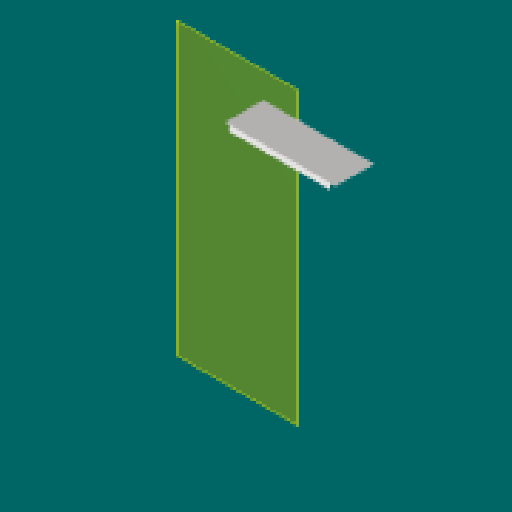
# Autodesk Inventor part: G_S
Saved by Autodesk Inventor 2023 (Build 270158000, 158)
## iProperties
Created: 2023-01-28
Part Number: G_S
Material: Generic
Document SubType Name: Sheet Metal
Designer: HeavyDrewno
Density: 1 g/cm^3
Sheet Metal Rule: Default
Appearance: Default
Author: HeavyDrewno
Autodesk Inventor part; units mm, degrees
ref_plane "YZ Plane" through (0, 0, 0) normal (1, 0, 0) x (0, 1, 0)
ref_plane "XZ Plane" through (0, 0, 0) normal (0, 1, 0) x (-1, 0, 0)
ref_plane "XY Plane" through (0, 0, 0) normal (0, 0, 1) x (1, 0, 0)
ref_plane "Work Plane1" through (0, 0, 0) normal (0, 0, 1) x (1, 0, 0)
sketch "Sketch1" plane through (0, 0, 0) normal (0, 0, 1) x (1, 0, 0)
  line L0 (-196, 470) -> (196, 470) construction
  line L1 (-196, 470) -> (-196, 330) construction
  line L2 (-196, 330) -> (196, 330)
  point P0 (0, 0)
  dimension "d0" = 140
  measures "d0" distance of L0.start L1.end
sketch "Sketch2" plane through (-196, 330, 136) normal (0, 0, 1) x (1, 0, 0)
  line L0 (16, 140) -> (16, -860) construction
  line L1 (376, 140) -> (376, -860) construction
  line L2 (0, 0) -> (392, 0)
  line L3 (16, 0) -> (16, -20)
  line L4 (16, -20) -> (376, -20)
  line L5 (376, -20) -> (376, 0)
  line L6 (16, 0) -> (376, 0)
  point P0 (196, -330)
  dimension "d12" = 20
  measures "d12" distance of L3.start L3.end
contour flange "Contour Flange1" sketch "Sketch1" thickness 2 bend radius 2 width 136 along (0, 0, 1) mid plane no both sides no wall seen from (0, 330, 0) lies toward (0, -1, 0) curves L2
bend "Bend1"
corner "Corner1"
sheet face with bend "Face1" sketch "Sketch2" thickness 2 toward (0, 0, 1) bend radius 2 relief straight relief width 2 relief depth 1
bend "Bend2"
equation "\"d1\" = Thickness"
equation "\"d2\" = BendReliefWidth"
equation "\"d3\" = BendReliefDepth"
equation "\"d4\" = MinimumRemnant"
equation "\"d5\" = TransitionRadius"
equation "\"d7\" = BendRadius"
equation "\"d9\" = CornerReliefSize"
equation "\"d10\" = GapSize"
equation "\"d11\" = JacobiRadiusSize"
equation "\"d13\" = BendRadius"
equation "\"d14\" = BendReliefWidth"
equation "\"d16\" = MinimumRemnant"
equation "\"d15\" = BendReliefDepth"
equation "\"d17\" = TransitionRadius"
equation "\"BendRadius\" = Thickness"
equation "\"BendReliefWidth\" = Thickness"
equation "\"BendReliefDepth\" = 0.5 * Thickness"
equation "\"CornerReliefSize\" = 4 * Thickness"
equation "\"MinimumRemnant\" = 2 * Thickness"
equation "\"TransitionRadius\" = BendRadius"
equation "\"JacobiRadiusSize\" = BendRadius"
equation "\"GapSize\" = Thickness"
equation "\"Thickness\" = 2"
body "Solid1"
